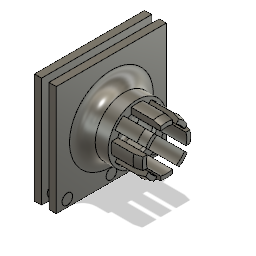
Houder 3e spiegel A v7 (Autodesk Fusion 360 design; units mm, degrees)
Autodesk Fusion 360 part; units mm, degrees
sketch "Sketch1" plane through (0, 0, 0) normal (1, 0, 0) x (0, 0, -1)
  circle A0 centre (0, 0) radius 7.1
  circle A1 centre (0, 0) radius 5.5
  circle A2 centre (0, 0) radius 6.3
  line L0 (-1.6, 5.2621) -> (-1.6, 6.9174)
  line L1 (0, 0) -> (0, 10.2823) construction
  line L2 (1.6, 5.2621) -> (1.6, 6.9174)
  circle A3 centre (0, 0) radius 7.9
  dimension "d1" = 14.2
  dimension "d3" = -1.6
  dimension "d5" = 1.6
  dimension "d14" = 0.8
  constraint coincident A0 L0.end
  constraint vertical L0
  constraint coincident A0.centre A1.centre
  constraint vertical L1
  constraint symmetric L0.start L1 L2.start
  constraint symmetric L0.end L1 L2.end
  constraint coincident A1 L0.start
  measures "d1" diameter of A0
  measures "d5" distance of L0 L1
extrude "Extrude2" add sketch "Sketch1" along normal blind 8 contours A0 A2 L0 L2 | A1 A2 L0 L2 picked at (-1.3355, 6.4197) picked at (1.3363, 5.5986) makes body 1
chamfer "Chamfer3" distance 0.5 distance2 2 1 edges at (8, 7.1, 0) measured on face at (8, 6.1959, 1.0713) on bodies 1
pattern_circular "C-Pattern1" count 8 over 360 about axis through (1.75, 0, 0) along (1, 0, 0) of bodies 1 makes body 2 at (5.3333, 3.4882, 4.2523) makes body 3 at (2.6667, 1.3393, 5.3344) makes body 4 at (2.6667, -2.825, 4.719) makes body 5 at (2.6667, -5.3344, 1.3393) makes body 6 at (5.3333, -4.0756, -3.6931) makes body 7 at (2.6667, -1.3393, -5.3344) makes body 8 at (5.3333, 4.2523, -3.4882)
extrude "Extrude3" add sketch "Sketch1" against normal blind 1 contours A0 A2 L0 L2 | A0 A2 L0 L2 | A1 A2 L0 L2 | A1 A2 L0 L2 | A3 bodies 1 2 3 4 5 6 7 8
sketch "Sketch2" plane through (-1, 0, 0) normal (-1, 0, 0) x (0, 0, 1)
  circle A0 centre (0, 0) radius 7.9
  circle A1 centre (0, 0) radius 7.1
  circle A2 centre (0, 0) radius 5.5
extrude "Extrude4" add sketch "Sketch2" along normal blind 6 contours A0 bodies 1
sketch "Sketch3" plane through (-7, 0, 0) normal (-1, 0, 0) x (0, 0, 1)
  circle A0 centre (0, 0) radius 7.1
  circle A1 centre (0, 0) radius 7.9
  line L0 (-15, -15) -> (15, -15)
  line L1 (15, -15) -> (15, 15)
  line L2 (15, 15) -> (-15, 15)
  line L3 (-15, 15) -> (-15, -15)
  line L4 (-15, -15) -> (15, 15) construction
  line L5 (15, -15) -> (-15, 15) construction
  dimension "d23" = 30
  dimension "d24" = 30
  constraint horizontal L0
  constraint perpendicular L0 L1
  constraint parallel L0 L2
  constraint parallel L1 L3
  constraint coincident L4 A0.centre
  constraint coincident L5 A0.centre
  constraint coincident A0.centre A1.centre
  measures "d23" distance of L1.end L2.end
  measures "d24" distance of L0.end L1.end
extrude "Extrude5" add sketch "Sketch3" along normal blind 2 contours A1 | L0 L1 L2 L3 bodies 1
fillet "Fillet1" radius 3.5 1 edges at (-7, -2.8568, -7.3654) on bodies 1
fillet "Fillet2" radius 3 1 edges at (-9, 2.5675, -6.6195) on bodies 1
sketch "Sketch4" plane through (-9, 0, 0) normal (-1, 0, 0) x (0, 0, 1)
  line L0 (-15, 15) -> (-15, -15)
  line L1 (-15, -15) -> (15, -15)
  line L2 (15, -15) -> (15, 15)
  line L3 (15, 15) -> (-15, 15)
  circle A0 centre (0, 0) radius 10.1
  circle A1 centre (0, -13) radius 1.45
  circle A2 centre (-12, -13) radius 1.45
  circle A3 centre (12, -13) radius 1.45
  dimension "d31" = 2.9
  dimension "d32" = 2
  dimension "d46" = 2.9
  dimension "d47" = 2.9
  dimension "d48" = 12
  dimension "d49" = 12
  constraint vertical A0.centre A1.centre
  constraint horizontal A1.centre A2.centre
  constraint horizontal A1.centre A3.centre
  measures "d31" diameter of A1
  measures "d32" distance of L1 A1.centre
  measures "d46" diameter of A2
  measures "d47" diameter of A3
  measures "d48" distance of A1.centre A3.centre
  measures "d49" distance of A1.centre A2.centre
extrude "Extrude6" cut sketch "Sketch4" against normal through all contours A1 | A2 | A3 bodies 1
ref_plane "WorkPlane1" through (-11, 0, 0) normal (-1, 0, 0) x (0, 0, 1)
sketch "Sketch5" plane through (-11, 0, 0) normal (-1, 0, 0) x (0, 0, -1)
  line L0 (15, -15) -> (-15, -15)
  line L1 (-15, -15) -> (-15, 15)
  line L2 (-15, 15) -> (15, 15)
  line L3 (15, 15) -> (15, -15)
  point P0 (15, -15)
  point P1 (-15, 15)
  constraint horizontal L0
  constraint vertical L1
  constraint horizontal L2
  constraint vertical L3
  constraint coincident P0 L0.start
  constraint coincident P1 L1.end
extrude "Extrude7" add sketch "Sketch5" along normal blind 2 separate body makes body 9
extrude "Extrude8" cut sketch "Sketch1" against normal up to surface (13 mm away) contours A1 bodies 9
copy_body "Body->Comp1" bodies 9 removing the originals makes body 10 in component "Component"
extrude "Extrude1" add sketch "Sketch4" against normal up to surface (4 mm away) from surface at 2 contours A1 | A2 | A3 bodies 10 in component "Component"
copy_body "Body->Comp2" bodies 1 removing the originals makes body 11 in component "Component'"
chamfer "Chamfer1" distance 1.6 distance2 5 1 edges at (-1, -2.5675, -6.6195) measured on face at (-1, -3.4839, 5.5312) on bodies 11 in component "Component'"
component "Component" placed x (1, 0, 0) y (0, 1, 0) z (0, 0, 1) at (0, 0, 0)
component "Component'" placed x (1, 0, 0) y (0, 1, 0) z (0, 0, 1) at (0, 0, 0)
equation "wall_thickness = 0.8 mm"
equation "d3 = -2 * wall_thickness"
equation "d4 = -wall_thickness"
equation "d5 = wall_thickness * 2"
equation "d14 = wall_thickness"
equation "d16 = -wall_thickness"
equation "d46 = d31"
equation "d47 = d31"
equation "d49 = d48"
